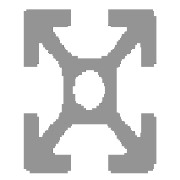
# Autodesk Inventor part: A3.3-MEM
Saved by Autodesk Inventor 2024 (Build 280153000, 153)
## iProperties
Created: 2024-03-14
Part Number: A3.3-MEM
Material: Generic
Description: A3.3
Document SubType Name: Modeling
Designer: Alex
Manufacturer: McMaster University
Language: en-US
Size Designation: 1
Categories: <MemberInstance><Categories><Category DisplayName="Structural Shapes" InternalName="089c4875-fa83-4c05-b084-43b9cc11f5ed" Mnemonic="GRDR"><CategoryParameter DisplayName="Mass per Length Unit" InternalName="0bb95a10-148f-4027-a459-38d7b056702a" Mnemonic="shpmass"/><CategoryParameter DisplayName="Section Area" InternalName="1ff91680-64b0-4202-b9a3-7fd3f94bba3b" Mnemonic="secarea"/><CategoryParameter DisplayName="Radius of Gyration (x)" InternalName="25778675-03e9-40c1-b6a8-4a9ed693320d" Mnemonic="gyrradx"/><CategoryParameter DisplayName="Torsional Rigidity Modulus" InternalName="26c1ec35-5026-4c63-ad0a-751cf684a536" Mnemonic="torrigmod"/><CategoryParameter DisplayName="Distance of the Center of Gravity X-X" InternalName="26c9bdb8-9c79-4b4f-a92e-8e197583c9c4" Mnemonic="grcendistX"/><CategoryParameter DisplayName="Legacy Member ID" InternalName="340afe4f-75d7-48d3-ab7d-943f3c3da468" Mnemonic="LegacyMemberID"/><CategoryParameter DisplayName="Base Length" InternalName="42e34263-8f20-4d0e-ad48-bf1385b87c24" Mnemonic="shplen"/><CategoryParameter DisplayName="Moment of Inertia (y)" InternalName="4b9f58ea-bced-460e-81ea-3d29ca5a49e3" Mnemonic="inermomy"/><CategoryParameter DisplayName="Moment of Inertia (x)" InternalName="4cd780bc-73d7-43ac-917a-579e5cbd684d" Mnemonic="inermomx"/><CategoryParameter DisplayName="Custom Base Point" InternalName="4f1d1b73-316d-484b-a3df-9cbabb16eb77" Mnemonic="shpBasePoint"/><CategoryParameter DisplayName="Shape Height" InternalName="50274e7d-5ac0-4796-92cb-c59e54983c67" Mnemonic="shpheig"/><CategoryParameter DisplayName="Section Module (y)" InternalName="59eaa5e9-d227-48dc-b6c1-6920f96e0f95" Mnemonic="secmody"/><CategoryParameter DisplayName="Section Designation" InternalName="5a64d034-428d-49c8-ba32-7619764de20f" Mnemonic="shpdes"/><CategoryParameter DisplayName="Section Module (x)" InternalName="72cfad18-cf51-4ed4-aaa7-c6b224f8419f" Mnemonic="secmodx"/><CategoryParameter DisplayName="Torsional Section Modulus" InternalName="7c55a8dc-8844-49f9-a867-cc677b30ec9a" Mnemonic="torsecmod"/><CategoryParameter DisplayName="Shape Width" InternalName="7c717d54-a18f-4666-b4d4-573cce22c62c" Mnemonic="shpwdth"/><CategoryParameter DisplayName="Second Shape Thickness" InternalName="9251a8e1-85fd-4e47-af99-afdb762317d9" Mnemonic="shpthick2"/><CategoryParameter DisplayName="FG Authored" InternalName="9c666724-f362-4ea7-ac62-f6a007de5c69" Mnemonic="shpFGAuto"/><CategoryParameter DisplayName="Distance of the Center of Gravity Y-Y" InternalName="bcc4fb17-7af4-436a-8f8c-d0aa3b0248c5" Mnemonic="grcendistY"/><CategoryParameter DisplayName="Radius of Gyration (y)" InternalName="bfa18ebe-1636-4dbe-8d42-b263e0b73184" Mnemonic="gyrrady"/><CategoryParameter DisplayName="Shape Thickness" InternalName="d109cf76-8eb4-42fc-9800-4409734adc67" Mnemonic="shpthick"/><CategoryParameter DisplayName="Coefficient of Shear Displacement" InternalName="de4c90c6-aaa8-468f-a335-6737b311b5d3" Mnemonic="shdispc"/><Category DisplayName="Square/Rectangular Tubes" InternalName="afc8e2d8-05d6-4609-8807-f98a9b7d2ed0" Mnemonic="SQRSHP"><CategoryParameter DisplayName="Section Area" InternalName="2f7f79dd-983c-4263-802a-5b6a1495fdc5" Mnemonic="secarea"/><CategoryParameter DisplayName="Section Module (x)" InternalName="50d965a6-04bf-46b9-8ace-861858d348e6" Mnemonic="secmodx"/><CategoryParameter DisplayName="Section Module (y)" InternalName="5106aeac-54a2-4159-a9af-8933dd39dba2" Mnemonic="secmody"/><CategoryParameter DisplayName="Shape Thickness" InternalName="52712fc5-f4ee-4eda-b3f2-6fce82c26419" Mnemonic="shpthick"/><CategoryParameter DisplayName="Moment of Inertia (y)" InternalName="55ec8510-8276-4c45-8f10-594e0fee7eb3" Mnemonic="inermomy"/><CategoryParameter DisplayName="Radius of Gyration (x)" InternalName="56c89926-a299-4389-a862-ac94c9691272" Mnemonic="gyrradx"/><CategoryParameter DisplayName="Radius" InternalName="5d8d062c-e28e-41c1-98da-8e5fee36da1a" Mnemonic="shprad"/><CategoryParameter DisplayName="Moment of Inertia (x)" InternalName="8c4637b6-6b69-4878-9d5d-26a32185d655" Mnemonic="inermomx"/><CategoryParameter DisplayName="Shape Width" InternalName="8c8a1782-5e80-4d77-858b-304b1c0ad1fd" Mnemonic="shpwdth"/><CategoryParameter DisplayName="Radius of Gyration (y)" InternalName="fa48a7f5-f030-40f9-a60b-de8a845b7104" Mnemonic="gyrrady"/></Category></Category><Category DisplayName="DataType" InternalName="23b78d0f-2648-40c6-8793-ca6db495c9e8" Mnemonic="DATATYPE"><CategoryParameter DisplayName="DisplayName" InternalName="05415f3d-3907-474b-a020-eb9d644f4cf3" Mnemonic="DISPLAYNAME"/><CategoryParameter DisplayName="Standard" InternalName="0c0a119c-1e12-4c84-803f-101930972f5e" Mnemonic="STANDARD"/><CategoryParameter DisplayName="Description" InternalName="13903e3d-64b1-4950-80da-f627842ea37f" Mnemonic="DESCRIPTION"/><CategoryParameter DisplayName="Designation" InternalName="2675968c-4ce5-49e0-a4f5-552d29089031" Mnemonic="DESIGNATION"/><CategoryParameter DisplayName="Default Row" InternalName="2af9ec52-faaa-4026-b378-f9fa4afca842" Mnemonic="DEFAULTROW"/><CategoryParameter DisplayName="Folder Name" InternalName="3f06958e-8713-4116-9be7-ed6184ecc97b" Mnemonic="FOLDERNAME"/><CategoryParameter DisplayName="Revision Guid" InternalName="45a75005-10b1-4dfc-8d6d-dfe629f0b93c" Mnemonic="REVISIONGUID"/><CategoryParameter DisplayName="FileName" InternalName="8b46a4cc-9585-4fed-90c3-899f57e09a73" Mnemonic="FILENAME"/><CategoryParameter DisplayName="StdsOrg" InternalName="8f5914e1-4693-403f-8ab5-d37768198c9d" Mnemonic="STDSORG"/><CategoryParameter DisplayName="Family Version" InternalName="914462f6-6e19-4b14-ba84-155b9680b1d0" Mnemonic="FAMILYREVISION"/><CategoryParameter DisplayName="Standard Revision" InternalName="91d5a463-65c2-4fde-b823-3b7fea5e8e17" Mnemonic="STANDARDREVISION"/><CategoryParameter DisplayName="Member Revision" InternalName="a65d44b9-392f-4f4f-857b-e4b3d54996fe" Mnemonic="MEMBERREVISION"/><CategoryParameter DisplayName="ClipFormat" InternalName="bc51e27b-3422-4e78-93ef-cec197ddf230" Mnemonic="CLIPFORMAT"/><CategoryParameter DisplayName="Manufacturer" InternalName="cd6c7a72-a28a-4e50-99a9-2c7f4e13e5ad" Mnemonic="MANUFACTURER"/><CategoryParameter DisplayName="InternalName" InternalName="cf1d0246-76d9-4b4a-8305-fa0409afb5c1" Mnemonic="INTERNALNAME"/><CategoryParameter DisplayName="IsMetric" InternalName="e2385c5b-1ea4-4823-96a8-8de651266ec3" Mnemonic="ISMETRIC"/><Category DisplayName="Part" InternalName="c0e0b642-3bcb-4cc8-9e80-f96d35c4afa4" Mnemonic="PART"><CategoryParameter DisplayName="Part Number" InternalName="016b6077-bfbe-49bd-92c9-d8d59c39c941" Mnemonic="PARTNUMBER"/><CategoryParameter DisplayName="Stock Number" InternalName="4dba7c1c-e26c-444e-836c-b08b433409a8" Mnemonic="STOCKNUMBER"/><CategoryParameter DisplayName="Material Key" InternalName="5c9a8adb-dd2b-4535-b97f-0a94a95fe41f" Mnemonic="MATERIALKEY"/><CategoryParameter DisplayName="Material" InternalName="818a152a-d3c3-49ca-80ee-df7d91421b8e" Mnemonic="MATERIAL"/></Category></Category></Categories><FamilyTemplate Id="A3.3"><FamilyTemplateParameters><FamilyTemplateParameter ObjectType="kUserParameterObject" ValueType="xs:double" Id="1" ObjectReferenceKey="Length"/><FamilyTemplateParameter ObjectType="kUserParameterObject" ValueType="xs:double" Id="3" ObjectReferenceKey="sigma"/><FamilyTemplateParameter ObjectType="kPartComponentDefinitionObject" ValueType="xs:string" Id="5" SubObjectId="Material"/><FamilyTemplateParameter ObjectType="kPropertyObject" ValueType="xs:string" Id="17" ObjectReferenceKey="{32853F0F-3444-11d1-9E93-0060B03C1CA6}" SubObjectId="5"/><FamilyTemplateParameter ObjectType="kPropertyObject" ValueType="xs:string" Id="18" ObjectReferenceKey="{32853F0F-3444-11d1-9E93-0060B03C1CA6}" SubObjectId="52"/></FamilyTemplateParameters></FamilyTemplate><CategoryParameterMap><ParamToTemplateMap><ParamToTemplate CategoryParameter="//CategoryParameter[@InternalName='cf1d0246-76d9-4b4a-8305-fa0409afb5c1']" ConstantValue="7a1cfee2-a943-4716-8884-d3571c99cc4f"/><ParamToTemplate CategoryParameter="//CategoryParameter[@InternalName='45a75005-10b1-4dfc-8d6d-dfe629f0b93c']" ConstantValue="4860a086-2cc3-4966-b2d1-6d7884aff654"/><ParamToTemplate CategoryParameter="//CategoryParameter[@InternalName='3f06958e-8713-4116-9be7-ed6184ecc97b']" ConstantValue="A3.3"/><ParamToTemplate CategoryParameter="//CategoryParameter[@InternalName='8f5914e1-4693-403f-8ab5-d37768198c9d']" TemplateParameter="10"/><ParamToTemplate CategoryParameter="//CategoryParameter[@InternalName='0c0a119c-1e12-4c84-803f-101930972f5e']" TemplateParameter="11"/><ParamToTemplate CategoryParameter="//CategoryParameter[@InternalName='91d5a463-65c2-4fde-b823-3b7fea5e8e17']" TemplateParameter="12"/><ParamToTemplate CategoryParameter="//CategoryParameter[@InternalName='cd6c7a72-a28a-4e50-99a9-2c7f4e13e5ad']" ConstantValue="McMaster University"/><ParamToTemplate CategoryParameter="//CategoryParameter[@InternalName='13903e3d-64b1-4950-80da-f627842ea37f']" ConstantValue="A3.3"/><ParamToTemplate CategoryParameter="//CategoryParameter[@InternalName='05415f3d-3907-474b-a020-eb9d644f4cf3']" ConstantValue="A3.3"/><ParamToTemplate CategoryParameter="//CategoryParameter[@InternalName='914462f6-6e19-4b14-ba84-155b9680b1d0']" ConstantValue="11"/><ParamToTemplate CategoryParameter="//CategoryParameter[@InternalName='bc51e27b-3422-4e78-93ef-cec197ddf230']" ConstantValue="CF_INVENTOR.STDPARTS"/><ParamToTemplate CategoryParameter="//CategoryParameter[@InternalName='e2385c5b-1ea4-4823-96a8-8de651266ec3']" ConstantValue="true"/><ParamToTemplate CategoryParameter="//CategoryParameter[@InternalName='2af9ec52-faaa-4026-b378-f9fa4afca842']" ConstantValue="1"/><ParamToTemplate CategoryParameter="//CategoryParameter[@InternalName='9c666724-f362-4ea7-ac62-f6a007de5c69']" ConstantValue="1"/><ParamToTemplate CategoryParameter="//CategoryParameter[@InternalName='8b46a4cc-9585-4fed-90c3-899f57e09a73']" ConstantValue="A3.3-MEM"/><ParamToTemplate CategoryParameter="//CategoryParameter[@InternalName='a65d44b9-392f-4f4f-857b-e4b3d54996fe']" ConstantValue="ec99d7c4-44db-43f0-8492-aa966c391349"/><ParamToTemplate CategoryParameter="//CategoryParameter[@InternalName='a65d44b9-392f-4f4f-857b-e4b3d54996fe']" ConstantValue="ec99d7c4-44db-43f0-8492-aa966c391349"/><ParamToTemplate CategoryParameter="//CategoryParameter[@InternalName='2675968c-4ce5-49e0-a4f5-552d29089031']" TemplateParameter="18"/><ParamToTemplate CategoryParameter="//CategoryParameter[@InternalName='42e34263-8f20-4d0e-ad48-bf1385b87c24']" TemplateParameter="1"/><ParamToTemplate CategoryParameter="//CategoryParameter[@InternalName='818a152a-d3c3-49ca-80ee-df7d91421b8e']" TemplateParameter="5"/><ParamToTemplate CategoryParameter="//CategoryParameter[@InternalName='016b6077-bfbe-49bd-92c9-d8d59c39c941']" TemplateParameter="17"/></ParamToTemplateMap></CategoryParameterMap></MemberInstance>
Density: 1 g/cm^3
Appearance: Default
IsCustomPart: 1
_CCFamilyMember: 1
_CCFamilyDisplayName: A3.3 - A3.3
_FrameMemberDoc: Frame Member File
_Version: 25.0.0
_GetPNFromCC: 1
Author: Alex
G_L: 129.938 mm
G_W: 20.000 mm
G_H: 20.000 mm
+ED99A0EE-E7E8-415B-812A-914AEDD657D7+CUTDETAIL1: Cut Angle 90.00 deg
+A98ACC74-E050-4F02-A194-219BD95E0743+CUTDETAIL2: Cut Angle 90.00 deg
Autodesk Inventor part; units mm, degrees
ref_plane "Start Plane" through (0, 0, 10.031) normal (0, 0, 1) x (1, 0, 0)
ref_plane "End Plane" through (0, 0, 139.969) normal (0, 0, 1) x (1, 0, 0)
sketch "Sketch" plane through (0, 0, 0) normal (0, 0, 1) x (1, 0, 0)
  line L0 (0, 0) -> (2.5, 0) construction
  line L1 (0, 0) -> (0, 2.5) construction
  line L2 (0, 4) -> (0, -4) construction
  line L3 (0, 4) -> (1.7574, 4)
  arc A0 (1.7574, 4) -> (3.1716, 4.5858) centre (1.7574, 6) ccw
  line L4 (3.1716, 4.5858) -> (5.7322, 7.1464)
  line L5 (-4, 0) -> (4, 0) construction
  line L6 (4, 0) -> (4, 1.7574)
  arc A1 (4.5858, 3.1716) -> (4, 1.7574) centre (6, 1.7574) ccw
  line L7 (4.5858, 3.1716) -> (7.1464, 5.7322)
  line L8 (0, 0) -> (10, 10) construction
  line L9 (0, 0) -> (19.6827, 0) construction
  arc A2 (8, 5.3787) -> (7.1464, 5.7322) centre (7.5, 5.3787) ccw
  line L10 (8, 5.3787) -> (8, 3.5)
  arc A3 (8, 3.5) -> (8.5, 3) centre (8.5, 3.5) ccw
  line L11 (8.5, 3) -> (9.5, 3)
  arc A4 (9.5, 3) -> (10, 3.5) centre (9.5, 3.5) ccw
  line L12 (10, 3.5) -> (10, 9)
  line L13 (10, 9) -> (10, 10) construction
  arc A5 (5.7322, 7.1464) -> (5.3787, 8) centre (5.3787, 7.5) ccw
  line L14 (5.3787, 8) -> (3.5, 8)
  arc A6 (3, 8.5) -> (3.5, 8) centre (3.5, 8.5) ccw
  line L15 (3, 8.5) -> (3, 9.5)
  arc A7 (3.5, 10) -> (3, 9.5) centre (3.5, 9.5) ccw
  line L16 (3.5, 10) -> (9, 10)
  arc A8 (10, 9) -> (9, 10) centre (9, 9) ccw
  line L17 (0, 4) -> (-1.7574, 4)
  arc A9 (-3.1716, 4.5858) -> (-1.7574, 4) centre (-1.7574, 6) ccw
  line L18 (-3.1716, 4.5858) -> (-5.7322, 7.1464)
  line L19 (-4, 0) -> (-4, 1.7574)
  arc A10 (-4, 1.7574) -> (-4.5858, 3.1716) centre (-6, 1.7574) ccw
  line L20 (-4.5858, 3.1716) -> (-7.1464, 5.7322)
  arc A11 (-7.1464, 5.7322) -> (-8, 5.3787) centre (-7.5, 5.3787) ccw
  line L21 (-8, 5.3787) -> (-8, 3.5)
  arc A12 (-8.5, 3) -> (-8, 3.5) centre (-8.5, 3.5) ccw
  line L22 (-8.5, 3) -> (-9.5, 3)
  arc A13 (-10, 3.5) -> (-9.5, 3) centre (-9.5, 3.5) ccw
  line L23 (-10, 3.5) -> (-10, 9)
  arc A14 (-5.3787, 8) -> (-5.7322, 7.1464) centre (-5.3787, 7.5) ccw
  line L24 (-5.3787, 8) -> (-3.5, 8)
  arc A15 (-3.5, 8) -> (-3, 8.5) centre (-3.5, 8.5) ccw
  line L25 (-3, 8.5) -> (-3, 9.5)
  arc A16 (-3, 9.5) -> (-3.5, 10) centre (-3.5, 9.5) ccw
  line L26 (-3.5, 10) -> (-9, 10)
  arc A17 (-9, 10) -> (-10, 9) centre (-9, 9) ccw
  line L27 (0, -4) -> (-1.7574, -4)
  arc A18 (-1.7574, -4) -> (-3.1716, -4.5858) centre (-1.7574, -6) ccw
  line L28 (-3.1716, -4.5858) -> (-5.7322, -7.1464)
  arc A19 (-5.7322, -7.1464) -> (-5.3787, -8) centre (-5.3787, -7.5) ccw
  line L29 (-5.3787, -8) -> (-3.5, -8)
  arc A20 (-3, -8.5) -> (-3.5, -8) centre (-3.5, -8.5) ccw
  line L30 (-3, -8.5) -> (-3, -9.5)
  arc A21 (-3.5, -10) -> (-3, -9.5) centre (-3.5, -9.5) ccw
  line L31 (-3.5, -10) -> (-9, -10)
  arc A22 (-10, -9) -> (-9, -10) centre (-9, -9) ccw
  line L32 (-10, -3.5) -> (-10, -9)
  arc A23 (-9.5, -3) -> (-10, -3.5) centre (-9.5, -3.5) ccw
  line L33 (-8.5, -3) -> (-9.5, -3)
  arc A24 (-8, -3.5) -> (-8.5, -3) centre (-8.5, -3.5) ccw
  line L34 (-8, -5.3787) -> (-8, -3.5)
  arc A25 (-8, -5.3787) -> (-7.1464, -5.7322) centre (-7.5, -5.3787) ccw
  line L35 (-4.5858, -3.1716) -> (-7.1464, -5.7322)
  arc A26 (-4.5858, -3.1716) -> (-4, -1.7574) centre (-6, -1.7574) ccw
  line L36 (-4, 0) -> (-4, -1.7574)
  line L37 (3.5, -10) -> (9, -10)
  arc A27 (9, -10) -> (10, -9) centre (9, -9) ccw
  line L38 (10, -3.5) -> (10, -9)
  arc A28 (10, -3.5) -> (9.5, -3) centre (9.5, -3.5) ccw
  line L39 (8.5, -3) -> (9.5, -3)
  arc A29 (8.5, -3) -> (8, -3.5) centre (8.5, -3.5) ccw
  line L40 (8, -5.3787) -> (8, -3.5)
  arc A30 (7.1464, -5.7322) -> (8, -5.3787) centre (7.5, -5.3787) ccw
  line L41 (4.5858, -3.1716) -> (7.1464, -5.7322)
  arc A31 (4, -1.7574) -> (4.5858, -3.1716) centre (6, -1.7574) ccw
  line L42 (4, 0) -> (4, -1.7574)
  line L43 (5.3787, -8) -> (3.5, -8)
  arc A32 (5.3787, -8) -> (5.7322, -7.1464) centre (5.3787, -7.5) ccw
  line L44 (3.1716, -4.5858) -> (5.7322, -7.1464)
  arc A33 (3.1716, -4.5858) -> (1.7574, -4) centre (1.7574, -6) ccw
  line L45 (0, -4) -> (1.7574, -4)
  arc A34 (3.5, -8) -> (3, -8.5) centre (3.5, -8.5) ccw
  line L46 (3, -8.5) -> (3, -9.5)
  arc A35 (3, -9.5) -> (3.5, -10) centre (3.5, -9.5) ccw
  circle A36 centre (0, 0) radius 2.5
  dimension "d1" = 8
  dimension "d2" = 2
  dimension "d3" = 8
  dimension "d4" = 2
  dimension "d5" = 2
  dimension "d7" = 45
  dimension "d8" = 0.5
  dimension "d9" = 0.5
  dimension "d10" = 0.5
  dimension "d12" = 2
  dimension "d17" = 7
  dimension "d18" = 10
  dimension "d19" = 0.5
  dimension "d20" = 1
  dimension "d21" = 0.5
  dimension "d22" = 0.5
  dimension "d23" = 2
  dimension "d24" = 7
  dimension "d25" = 5
  constraints: 94 end point, 81 symmetric about line, 72 point on circle, 37 centre point, 18 tangent, 6 horizontal, 5 vertical, 3 parallel, 2 coincident, 2 equal length, 2 midpoint, 2 perpendicular, 27 other
  measures "d1" distance of L2.start L2.end
  measures "d2" radius of A0
  measures "d3" distance of L5.start L5.end
  measures "d4" radius of A1
  measures "d5" distance between parallel lines of L7 L4
  measures "d7" angle of L9 L8
  measures "d8" radius of A2
  measures "d9" radius of A3
  measures "d10" radius of A4
  measures "d12" distance between parallel lines of L12 L10
  measures "d17" distance from line of L8.end L11
  measures "d18" distance from line of L8.end L9
  measures "d19" radius of A5
  measures "d20" radius of A8
  measures "d21" radius of A7
  measures "d22" radius of A6
  measures "d23" distance between parallel lines of L14 L16
  measures "d24" distance between parallel lines of L12 L15
  measures "d25" diameter of A36
extrude "Body" add sketch "Sketch" along normal up to surface (129.938 mm away) from surface at 10.031
sketch "Sketch6" plane through (0, 0, 0) normal (0, 0, 1) x (1, 0, 0)
  line L0 (0, 0) -> (10, 0)
ref_plane "Work Plane5" through (0, 0, 0) normal (0, -1, 0) x (1, 0, 0)
sketch "Sketch7" plane through (0, 0, 0) normal (0, -1, 0) x (1, 0, 0)
  line L0 (-2, 10.031) -> (12, 10.031)
  line L1 (-2, 139.969) -> (12, 139.969)
  dimension "d33" = 129.938
  measures "d33" distance between parallel lines of L0 L1
ref_plane "Work Plane6" through (200, 9, 139.969) normal (0, 0, 1) x (1, 0, 0)
split "Split1" plane through (200, 9, 139.969) removes the side toward (0, 0, 1)
ref_plane "Work Plane7" through (-300, 9, 10.031) normal (0, 0, -1) x (-1, 0, 0)
split "Split2" plane through (-300, 9, 10.031) removes the side toward (0, 0, -1)
equation "\"d1\" = 8 * sigma"
equation "\"d2\" = 2 * sigma"
equation "\"d3\" = 8 * sigma"
equation "\"d4\" = 2 * sigma"
equation "\"d5\" = 2 * sigma"
equation "\"d8\" = 0.5 * sigma"
equation "\"d9\" = 0.5 * sigma"
equation "\"d10\" = 0.5 * sigma"
equation "\"d12\" = 2 * sigma"
equation "\"d17\" = 7 * sigma"
equation "\"d18\" = sigma"
equation "\"d19\" = 0.5 * sigma"
equation "\"d20\" = sigma"
equation "\"d21\" = 0.5 * sigma"
equation "\"d22\" = 0.5 * sigma"
equation "\"d23\" = 2 * sigma"
equation "\"d24\" = 7 * sigma"
equation "\"d25\" = 5 * sigma"
equation "\"sigma\" = 1"
equation "\"G_OFFSET_START\" = -10.031"
equation "\"G_OFFSET_END\" = -10.031"
equation "\"d28\" = -G_OFFSET_START"
equation "\"d29\" = Length + G_OFFSET_END"
equation "\"G_L\" = d33"
equation "\"Length\" = 150"
body "Solid1"
